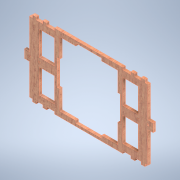
# Autodesk Inventor part: DoorFrameRear_V2
Saved by Autodesk Inventor 2022.2 (Build 262287000, 287)
## iProperties
Created: 2023-03-04
Part Number: DoorFrameRear_V2
Material: Wood (Oak)
Document SubType Name: Modeling
Designer: jaege
Density: 0.76 g/cm^3
Appearance: Red Oak - Natural Low Gloss
Author: jaege
Autodesk Inventor part; units mm, degrees
ref_plane "YZ Plane" through (0, 0, 0) normal (1, 0, 0) x (0, 1, 0)
ref_plane "XZ Plane" through (0, 0, 0) normal (0, 1, 0) x (-1, 0, 0)
ref_plane "XY Plane" through (0, 0, 0) normal (0, 0, 1) x (1, 0, 0)
sketch "Sketch1" plane through (0, 0, 0) normal (0, 0, 1) x (1, 0, 0)
  line L0 (45, -50) -> (-45, -50)
  line L1 (-45, -50) -> (-45, 50)
  line L2 (-45, 50) -> (45, 50)
  line L3 (45, 50) -> (45, -50)
  line L4 (45, -50) -> (-45, 50) construction
  line L5 (-45, -50) -> (45, 50) construction
  line L6 (53, 58) -> (-53, 58)
  line L7 (-53, 58) -> (-53, 54.5)
  line L8 (-53, -58) -> (53, -58)
  line L9 (53, -58) -> (53, -54.5)
  line L10 (-20, 50) -> (20, 50)
  line L11 (20, 50) -> (20, 54)
  line L12 (20, 54) -> (-20, 54)
  line L13 (-20, 54) -> (-20, 50)
  line L14 (-20, -50) -> (20, -50)
  line L15 (20, -50) -> (20, -54)
  line L16 (20, -54) -> (-20, -54)
  line L17 (-20, -54) -> (-20, -50)
  line L18 (-45, 20) -> (-49, 20)
  line L19 (-49, 20) -> (-49, -20)
  line L20 (-49, -20) -> (-45, -20)
  line L21 (-45, -20) -> (-45, 20)
  line L22 (45, 20) -> (49, 20)
  line L23 (49, 20) -> (49, -20)
  line L24 (49, -20) -> (45, -20)
  line L25 (45, -20) -> (45, 20)
  line L26 (-53, 6.5) -> (-77, 6.5)
  line L27 (-100, 6.5) -> (-100, -6.5)
  line L28 (-100, -6.5) -> (-92, -6.5)
  line L29 (-53, -6.5) -> (-53, 6.5) construction
  line L30 (-53, 0) -> (53, 0)
  circle A0 centre (-92, 0) radius 1.45
  circle A1 centre (-77, 0) radius 1.45
  line L31 (0, 50) -> (0, -50)
  line L32 (-53, 6.5) -> (-53, -6.5) construction
  line L33 (-53, -6.5) -> (-53, -44.5)
  line L34 (53, 6.5) -> (53, 44.5)
  line L35 (53, -6.5) -> (53, 6.5) construction
  line L36 (-92, -6.5) -> (-77, -6.5) construction
  line L37 (-77, -6.5) -> (-77, -44.5)
  line L38 (-77, -58) -> (-92, -58) construction
  line L39 (-92, -58) -> (-92, -54.5) construction
  line L40 (-92, -58) -> (-77, -58) construction
  line L41 (-77, -58) -> (-77, -58.5) construction
  line L42 (-77, -58.5) -> (-81.5, -58.5) construction
  line L43 (-92, -58.5) -> (-92, -58) construction
  line L44 (-92, -54.5) -> (-87.5, -54.5)
  line L45 (-87.5, -54.5) -> (-87.5, -58.5)
  line L46 (-81.5, -58.5) -> (-81.5, -54.5)
  line L47 (-81.5, -54.5) -> (-77, -54.5)
  line L48 (-77, 6.5) -> (-77, 44.5)
  line L49 (-77, 58) -> (-92, 58) construction
  line L50 (-92, 58) -> (-92, 54.5) construction
  line L51 (-92, 58) -> (-77, 58) construction
  line L52 (-77, 58) -> (-77, 58.5) construction
  line L53 (-77, 58.5) -> (-81.5, 58.5) construction
  line L54 (-92, 58.5) -> (-92, 58) construction
  line L55 (-92, 54.5) -> (-87.5, 54.5)
  line L56 (-87.5, 54.5) -> (-87.5, 58.5)
  line L57 (-81.5, 58.5) -> (-81.5, 54.5)
  line L58 (-81.5, 54.5) -> (-77, 54.5)
  line L59 (-77, 6.5) -> (-92, 6.5) construction
  line L60 (-92, 6.5) -> (-100, 6.5)
  line L61 (-92, -6.5) -> (-77, -6.5) construction
  line L62 (-77, -6.5) -> (-53, -6.5)
  line L63 (-77, 54.5) -> (-77, 58) construction
  line L64 (-92, 54.5) -> (-92, 6.5)
  line L65 (-87.5, 58.5) -> (-92, 58.5) construction
  line L66 (-81.5, 58.5) -> (-87.5, 58.5)
  line L67 (-92, -54.5) -> (-92, -6.5)
  line L68 (-87.5, -58.5) -> (-92, -58.5) construction
  line L69 (-81.5, -58.5) -> (-87.5, -58.5)
  line L70 (-77, -54.5) -> (-77, -58) construction
  line L71 (-77, 54.5) -> (-71.5, 54.5)
  line L72 (-53, 54.5) -> (-53, 44.5) construction
  line L73 (-53, 44.5) -> (-77, 44.5)
  line L74 (-77, 44.5) -> (-77, 54.5) construction
  line L75 (-77, -54.5) -> (-71.5, -54.5)
  line L76 (-53, -54.5) -> (-53, -54)
  line L77 (-53, -44.5) -> (-77, -44.5)
  line L78 (-77, -44.5) -> (-77, -54.5) construction
  line L79 (-71.5, 54.5) -> (-65.5, 54.5) construction
  line L80 (-65.5, 54.5) -> (-65.5, 58.5)
  line L81 (-65.5, 58.5) -> (-71.5, 58.5)
  line L82 (-71.5, 58.5) -> (-71.5, 54.5)
  line L83 (-71.5, -54.5) -> (-65.5, -54.5) construction
  line L84 (-65.5, -54.5) -> (-65.5, -58.5)
  line L85 (-65.5, -58.5) -> (-71.5, -58.5)
  line L86 (-71.5, -58.5) -> (-71.5, -54.5)
  line L87 (-71.5, 54.5) -> (-65.5, 54.5) construction
  line L88 (-65.5, 54.5) -> (-53, 54.5)
  line L89 (-77, 44.5) -> (-77, 54.5) construction
  line L90 (-53, 44.5) -> (-53, 6.5)
  line L91 (-53, 54.5) -> (-53, 44.5) construction
  line L92 (-77, -44.5) -> (-77, -54.5) construction
  line L93 (-53, -44.5) -> (-53, -54.5) construction
  line L94 (-53, -54) -> (-53, -44.5) construction
  line L95 (-65.5, -54.5) -> (-53, -54.5)
  line L96 (-71.5, -54.5) -> (-65.5, -54.5) construction
  line L97 (-53, -54.5) -> (-53, -58)
  line L98 (53, 6.5) -> (77, 6.5)
  line L99 (100, 6.5) -> (100, -6.5)
  line L100 (100, -6.5) -> (92, -6.5)
  circle A2 centre (92, 0) radius 1.45
  circle A3 centre (77, 0) radius 1.45
  line L101 (92, -6.5) -> (77, -6.5) construction
  line L102 (77, -6.5) -> (77, -44.5)
  line L103 (77, -58) -> (92, -58) construction
  line L104 (92, -58) -> (92, -54.5) construction
  line L105 (92, -58) -> (77, -58) construction
  line L106 (77, -58) -> (77, -58.5) construction
  line L107 (77, -58.5) -> (81.5, -58.5) construction
  line L108 (92, -58.5) -> (92, -58) construction
  line L109 (92, -54.5) -> (87.5, -54.5)
  line L110 (87.5, -54.5) -> (87.5, -58.5)
  line L111 (81.5, -58.5) -> (81.5, -54.5)
  line L112 (81.5, -54.5) -> (77, -54.5)
  line L113 (92, 54.5) -> (87.5, 54.5)
  line L114 (92, 58) -> (92, 54.5) construction
  line L115 (77, 6.5) -> (77, 44.5)
  line L116 (81.5, 54.5) -> (77, 54.5)
  line L117 (77, 58) -> (92, 58) construction
  line L118 (92, 58) -> (77, 58) construction
  line L119 (77, 58) -> (77, 58.5) construction
  line L120 (77, 58.5) -> (81.5, 58.5) construction
  line L121 (81.5, 58.5) -> (81.5, 54.5)
  line L122 (92, 58.5) -> (92, 58) construction
  line L123 (87.5, 54.5) -> (87.5, 58.5)
  line L124 (77, 6.5) -> (92, 6.5) construction
  line L125 (92, 6.5) -> (100, 6.5)
  line L126 (92, -6.5) -> (77, -6.5) construction
  line L127 (77, -6.5) -> (53, -6.5)
  line L128 (77, 54.5) -> (77, 58) construction
  line L129 (92, 54.5) -> (92, 6.5)
  line L130 (87.5, 58.5) -> (92, 58.5) construction
  line L131 (81.5, 58.5) -> (87.5, 58.5)
  line L132 (92, -54.5) -> (92, -6.5)
  line L133 (87.5, -58.5) -> (92, -58.5) construction
  line L134 (81.5, -58.5) -> (87.5, -58.5)
  line L135 (77, -54.5) -> (77, -58) construction
  line L136 (77, 54.5) -> (71.5, 54.5)
  line L137 (53, 44.5) -> (77, 44.5)
  line L138 (77, 44.5) -> (77, 54.5) construction
  line L139 (77, -54.5) -> (71.5, -54.5)
  line L140 (53, -44.5) -> (77, -44.5)
  line L141 (77, -44.5) -> (77, -54.5) construction
  line L142 (71.5, 54.5) -> (65.5, 54.5) construction
  line L143 (65.5, 54.5) -> (65.5, 58.5)
  line L144 (65.5, 58.5) -> (71.5, 58.5)
  line L145 (71.5, 58.5) -> (71.5, 54.5)
  line L146 (71.5, -54.5) -> (65.5, -54.5) construction
  line L147 (65.5, -54.5) -> (65.5, -58.5)
  line L148 (65.5, -58.5) -> (71.5, -58.5)
  line L149 (71.5, -58.5) -> (71.5, -54.5)
  line L150 (71.5, 54.5) -> (65.5, 54.5) construction
  line L151 (65.5, 54.5) -> (53, 54.5)
  line L152 (77, 44.5) -> (77, 54.5) construction
  line L153 (77, -44.5) -> (77, -54.5) construction
  line L154 (65.5, -54.5) -> (53, -54.5)
  line L155 (71.5, -54.5) -> (65.5, -54.5) construction
  line L156 (53, 44.5) -> (53, 54.5) construction
  line L157 (53, 54.5) -> (53, 58)
  line L158 (53, -44.5) -> (53, -6.5)
  line L159 (53, -54.5) -> (53, -44.5) construction
  point P0 (0, 0)
  point P1 (0, 54)
  point P2 (0, 0)
  point P3 (-49, 0)
  point P4 (0, 0)
  point P5 (-53, 0)
  point P6 (0, 0)
  point P7 (0, 0)
  point P8 (-84.5, -58)
  point P9 (-84.5, 58)
  point P10 (-65, 44.5)
  point P11 (-81.5, 56.5)
  point P12 (-71.5, 56.5)
  point P13 (84.5, -58)
  point P14 (84.5, 58)
  point P15 (65, 44.5)
  point P16 (81.5, 56.5)
  point P17 (71.5, 56.5)
  dimension "d0" = 100
  dimension "d1" = 90
  dimension "d2" = 8
  dimension "d3" = 4
  dimension "d4" = 4
  dimension "d5" = 40
  dimension "d6" = 40
  dimension "d7" = 4
  dimension "d8" = 4
  dimension "d9" = 13
  dimension "d10" = 47
  dimension "d11" = 2.9
  dimension "d12" = 15
  dimension "d13" = 24
  dimension "d14" = 4
  dimension "d15" = 4
  dimension "d16" = 15
  dimension "d17" = 0.5
  dimension "d18" = 6
  dimension "d19" = 4.5
  dimension "d20" = 4.5
  dimension "d21" = 4
  dimension "d24" = 10
  dimension "d25" = 10
  dimension "d27" = 10
  dimension "d28" = 6
  constraints: 320 end point, 95 parallel, 62 symmetric about line, 33 perpendicular, 18 horizontal, 16 midpoint, 16 point on line, 7 horizontal alignment, 5 vertical alignment, 4 centre point, 1 collinear, 1 equal radius, 3 other
  measures "d0" distance of L0.end L1.end
  measures "d1" distance of L1.end L2.end
  measures "d2" distance between parallel lines of L2 L6
  measures "d3" distance of L10.end L11.end
  measures "d4" distance of L14.end L15.end
  measures "d5" distance of L11.end L12.end
  measures "d6" distance of L22.end L23.end
  measures "d7" distance of L22.start L22.end
  measures "d8" distance of L18.start L18.end
  measures "d9" distance of L27.start L27.end
  measures "d10" distance of L26.start L27.start
  measures "d11" diameter of A0
  measures "d12" distance of A1.centre A0.centre
  measures "d13" distance from line of L7 A1.centre
  measures "d14" distance between parallel lines of L16 L8
  measures "d15" distance between parallel lines of L33 L19
  measures "d16" distance of L38.start L38.end
  measures "d17" distance of L38.start L41.end
  measures "d18" distance between parallel lines of L46 L45
  measures "d19" distance of L46.end L47.end
  measures "d20" distance of L39.end L44.end
  measures "d21" distance of L44.end L45.end
  measures "d24" distance from line of point (-65, 44.5) L71
  measures "d25" distance between parallel lines of L77 L75
  measures "d27" distance of L85.end L42.end
  measures "d28" distance of L84.end L85.end
extrude "Extrusion1" add sketch "Sketch1" along normal blind 4
body "Solid1"
